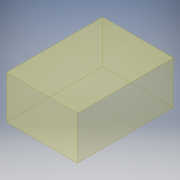
# Autodesk Inventor part: case
Saved by Autodesk Inventor 2019 (Build 230136000, 136)
## iProperties
Created: 2020-03-14
Part Number: case
Material: Generic
Document SubType Name: Modeling
Designer: james
Density: 1 g/cm^3
Appearance: Clear - Yellow
Author: james
Autodesk Inventor part; units mm, degrees
ref_plane "YZ Plane" through (0, 0, 0) normal (1, 0, 0) x (0, 1, 0)
ref_plane "XZ Plane" through (0, 0, 0) normal (0, 1, 0) x (-1, 0, 0)
ref_plane "XY Plane" through (0, 0, 0) normal (0, 0, 1) x (1, 0, 0)
sketch "Sketch1" plane through (0, 0, 0) normal (0, 1, 0) x (-1, 0, 0)
  line L0 (247.2692, 231.1318) -> (-108.3308, 231.1318)
  line L1 (-108.3308, 231.1318) -> (-108.3308, -251.4682)
  line L2 (-108.3308, -251.4682) -> (247.2692, -251.4682)
  line L3 (247.2692, -251.4682) -> (247.2692, 231.1318)
  point P0 (0, 0)
  dimension "d0" = 482.6
  dimension "d1" = 355.6
  constraints: 8 end point, 2 parallel, 1 horizontal, 1 perpendicular
  measures "d0" distance of L0.end L1.end
  measures "d1" distance of L0.start L0.end
extrude "Extrusion1" add sketch "Sketch1" along normal blind 215.9
body "Solid1"
